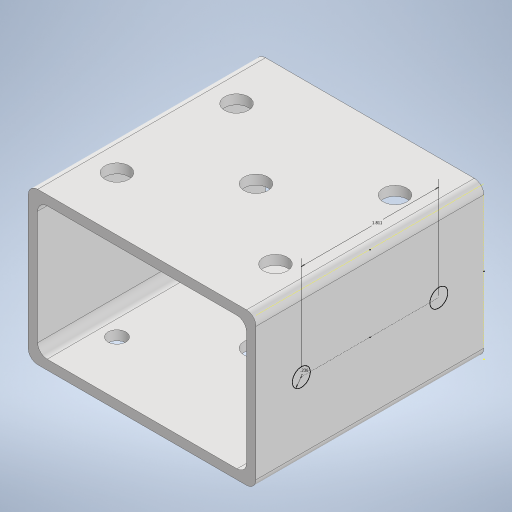
# Autodesk Inventor part: 2x3_Tube
Saved by Autodesk Inventor 2023 (Build 270158000, 158)
## iProperties
Created: 2022-05-03
Part Number: 2x3_Tube
Material: Generic
Document SubType Name: Modeling
Designer: plebbb
Density: 1 g/cm^3
Appearance: Default
Mass: 57.0623 g
Surface Area: 373.644 cm^2
Volume: 57.0623 cm^3
Author: plebbb
Autodesk Inventor part; units mm, degrees
ref_plane "YZ Plane" through (0, 0, 0) normal (1, 0, 0) x (0, 1, 0)
ref_plane "XZ Plane" through (0, 0, 0) normal (0, 1, 0) x (-1, 0, 0)
ref_plane "XY Plane" through (0, 0, 0) normal (0, 0, 1) x (1, 0, 0)
sketch "Sketch1" plane through (0, 0, 0) normal (0, 0, 1) x (1, 0, 0)
  line L0 (0, 0) -> (76.2, 0)
  line L1 (76.2, 0) -> (76.2, 50.8)
  line L2 (76.2, 50.8) -> (0, 50.8)
  line L3 (0, 50.8) -> (0, 0)
  dimension "d0" = 76.2
  dimension "d1" = 50.8
  constraints: 8 end point, 2 parallel, 1 horizontal, 1 perpendicular
  measures "d0" distance of L1.end L2.end
  measures "d1" distance of L0.end L1.end
extrude "Extrusion1" add sketch "Sketch1" along normal blind 76.2
shell "Shell1" thickness 3.175 removed faces 2 at (50.8, 16.9333, 76.2) at (50.8, 16.9333, 0)
sketch "Sketch2" plane through (0, 0, 0) normal (0, -1, 0) x (1, 0, 0)
  line L0 (11.6, 18.1) -> (64.6, 18.1) construction
  line L1 (64.6, 18.1) -> (64.6, 58.1) construction
  line L2 (64.6, 58.1) -> (11.6, 58.1) construction
  line L3 (11.6, 58.1) -> (11.6, 18.1) construction
  circle A0 centre (11.6, 18.1) radius 3
  circle A1 centre (11.6, 58.1) radius 3
  circle A2 centre (64.6, 58.1) radius 3
  circle A3 centre (64.6, 18.1) radius 3
  line L4 (0, 0) -> (0, 76.2) construction
  line L5 (0, 0) -> (76.2, 0) construction
  point P0 (11.6, 38.1)
  point P1 (0, 38.1)
  point P2 (38.1, 18.1)
  point P3 (38.1, 0)
  dimension "d5" = 6
  dimension "d6" = 53
  dimension "d7" = 40
  constraints: 8 end point, 4 centre point, 4 coincident, 4 midpoint, 3 equal radius, 2 parallel, 1 horizontal, 1 horizontal alignment, 1 perpendicular, 1 vertical alignment
  measures "d5" diameter of A0
  measures "d6" distance of L1.end L2.end
  measures "d7" distance of L2.end L0.start
extrude "Extrusion2" cut sketch "Sketch2" against normal blind 101.6
sketch "Sketch3" plane through (0, 50.8, 0) normal (0, 1, 0) x (1, 0, 0)
  line L0 (76.2, 0) -> (0, 0) construction
  line L1 (0, 0) -> (0, -76.2) construction
  circle A0 centre (38.1, -38.1) radius 4
  point P0 (38.1, 0)
  point P1 (0, -38.1)
  dimension "d10" = 8
  constraints: 2 midpoint, 1 centre point, 1 horizontal alignment, 1 vertical alignment
  measures "d10" diameter of A0
extrude "Extrusion3" cut sketch "Sketch3" against normal blind 101.6
fillet "Fillet1" radius 3.175 8 edges at (0, 50.8, 38.1) (76.2, 50.8, 38.1) (0, 0, 38.1) (73.025, 3.175, 38.1) (73.025, 47.625, 38.1) (76.2, 0, 38.1) (3.175, 47.625, 38.1) (3.175, 3.175, 38.1)
sketch "Sketch4" plane through (3.175, 50.8, 0) normal (0, 1, 0) x (1, 0, 0)
  circle A0 centre (8.425, -18.1) radius 4
  circle A1 centre (8.425, -58.1) radius 4
  circle A2 centre (61.425, -18.1) radius 4
  circle A3 centre (61.425, -58.1) radius 4
  circle A4 centre (8.425, -18.1) radius 3 construction
  circle A5 centre (61.425, -18.1) radius 3 construction
  circle A6 centre (8.425, -58.1) radius 3 construction
  circle A7 centre (61.425, -58.1) radius 3 construction
  point P0 (-3.175, 0)
  dimension "d14" = 8
  constraints: 4 centre point, 4 concentric, 3 equal radius
  measures "d14" diameter of A0
extrude "Extrusion4" cut sketch "Sketch4" against normal up to surface (3.175 mm away)
sketch "Sketch5" plane through (76.2, 3.175, 0) normal (1, 0, 0) x (0, 0, -1)
  circle A0 centre (-61.1, 22.225) radius 3
  circle A1 centre (-15.1, 22.225) radius 3
  line L0 (-61.1, 22.225) -> (-15.1, 22.225) construction
  line L1 (-62.1, 47.625) -> (-54.1, 47.625) construction
  line L2 (-22.1, 47.625) -> (-14.1, 47.625) construction
  line L3 (-62.1, 47.625) -> (-54.1, 47.625) construction
  line L4 (-22.1, 47.625) -> (-14.1, 47.625) construction
  line L5 (-42.1, 47.625) -> (-34.1, 47.625) construction
  line L6 (0, 47.625) -> (-76.2, 47.625) construction
  line L7 (-76.2, 47.625) -> (0, 47.625) construction
  line L8 (0, 0) -> (0, 44.45) construction
  point P0 (0, -3.175)
  point P1 (-38.1, 47.625)
  point P2 (-38.1, 22.225)
  point P3 (0, 22.225)
  dimension "d17" = 6
  dimension "d18" = 46
  constraints: 3 midpoint, 2 centre point, 2 end point, 1 coincident, 1 equal radius, 1 horizontal, 1 horizontal alignment, 1 vertical alignment
  measures "d17" diameter of A0
  measures "d18" distance of L0.start L0.end
body "Solid1"
